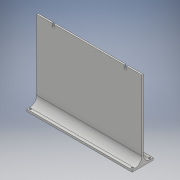
# Autodesk Inventor part: apriltag_body
Saved by Autodesk Inventor 2018 (Build 220112000, 112)
## iProperties
Created: 2020-02-24
Part Number: apriltag_body
Material: Generic
Document SubType Name: Modeling
Designer: bitbots
Density: 1 g/cm^3
Appearance: Default
Author: bitbots
Autodesk Inventor part; units mm, degrees
ref_plane "YZ Plane" through (0, 0, 0) normal (1, 0, 0) x (0, 1, 0)
ref_plane "XZ Plane" through (0, 0, 0) normal (0, 1, 0) x (-1, 0, 0)
ref_plane "XY Plane" through (0, 0, 0) normal (0, 0, 1) x (1, 0, 0)
sketch "Sketch1" plane through (0, 0, 0) normal (0, 1, 0) x (-1, 0, 0)
  line L0 (75, 55) -> (-75, 55)
  line L1 (-75, 55) -> (-75, -55)
  line L2 (-75, -55) -> (75, -55)
  line L3 (75, -55) -> (75, 55)
  line L4 (75, 55) -> (-75, -55) construction
  line L5 (-75, 55) -> (75, -55) construction
  point P0 (0, 0)
  dimension "d0" = 150
  dimension "d1" = 110
  constraints: 12 end point, 2 midpoint, 2 parallel, 1 horizontal, 1 perpendicular
  measures "d0" distance of L2.end L1.end
  measures "d1" distance of L1.end L0.end
extrude "Extrusion1" add sketch "Sketch1" along normal blind 2
sketch "Sketch2" plane through (75, 0, -55) normal (0, 0, -1) x (-1, 0, 0)
  line L0 (0, 0) -> (150, 0) projected
  line L1 (150, 0) -> (150, 2) projected
  line L2 (0, 2) -> (150, 2) projected
  line L3 (0, 0) -> (0, 2) projected
  line L4 (0, 0) -> (0, 2) construction
  line L5 (0, 0) -> (150, 2) construction
  line L6 (150, 0) -> (0, 0) construction
  line L7 (150, 0) -> (0, 2) construction
  line L8 (150, -14) -> (0, -14)
  line L9 (0, -14) -> (0, 16)
  line L10 (0, 16) -> (150, 16)
  line L11 (150, 16) -> (150, -14)
  line L12 (150, -14) -> (0, 16) construction
  line L13 (0, -14) -> (150, 16) construction
  point P0 (75, 0)
  point P1 (75, 1)
  dimension "d4" = 30
  dimension "d5" = 150
  constraints: 16 end point, 3 midpoint, 2 parallel, 1 horizontal, 1 perpendicular
  measures "d4" distance of L8.end L9.end
  measures "d5" distance between parallel lines of L11 L9
extrude "Extrusion2" add sketch "Sketch2" along normal blind 3
fillet "Fillet1" radius 10 2 edges at (0, 0, -55) (0, 2, -55)
sketch "Sketch3" plane through (0, 0, 0) normal (0, -1, 0) x (1, 0, 0)
  line L0 (0, 0) -> (0, 5)
  line L1 (0, 0) -> (5, 0) construction
  line L2 (-50, 55) -> (50, 55)
  line L3 (50, 55) -> (50, -45)
  line L4 (50, -45) -> (-50, -45)
  line L5 (-50, -45) -> (-50, 55)
  line L6 (-50, 55) -> (50, -45) construction
  line L7 (50, 55) -> (-50, -45) construction
  line L8 (-50, 55) -> (-53, 55)
  line L9 (-53, 55) -> (-53, 50)
  line L10 (-53, 50) -> (-50, 50)
  line L11 (-50, 50) -> (-50, 55)
  line L12 (50, 55) -> (53, 55)
  line L13 (53, 55) -> (53, 50)
  line L14 (53, 50) -> (50, 50)
  line L15 (50, 50) -> (50, 55)
  dimension "d9" = 5
  dimension "d10" = 90
  dimension "d11" = 100
  dimension "d12" = 100
  dimension "d13" = 3
  dimension "d14" = 5
  dimension "d15" = 3
  dimension "d16" = 5
  constraints: 32 end point, 6 parallel, 4 horizontal, 4 perpendicular, 2 midpoint, 1 vertical
  measures "d9" distance of L0.start L0.end
  measures "d10" angle of L1 L0
  measures "d11" distance of L3.end L4.end
  measures "d12" distance of L2.end L3.end
  measures "d13" distance of L10.end L9.end
  measures "d14" distance of L9.end L8.end
  measures "d15" distance of L13.end L14.end
  measures "d16" distance of L12.end L13.end
extrude "Extrusion3" cut sketch "Sketch3" against normal up to surface (2 mm away) contours L5 L10 L9 L8 | L12 L13 L14 L3
sketch "Sketch4" plane through (75, 0, -58) normal (0, 0, -1) x (-1, 0, 0)
  line L0 (75, 0) -> (147.5, 0)
  line L1 (0, 0) -> (150, 0) projected
  line L2 (75, 0) -> (147.5, 0) construction
  line L3 (147.5, 0) -> (147.5, -11.5)
  line L4 (150, -10) -> (0, -10) projected
  circle A0 centre (147.5, -11.5) radius 1.35
  line L5 (75, 0) -> (75, -10)
  line L6 (75, 0) -> (85, 0) construction
  circle A1 centre (147.5, 13.5) radius 1.35
  circle A2 centre (2.5, -11.5) radius 1.35
  circle A3 centre (2.5, 13.5) radius 1.35
  line L7 (150, 2) -> (0, 2) projected
  line L8 (75, 0) -> (75, 1)
  line L9 (75, 0) -> (76, 0) construction
  dimension "d19" = 72.5
  dimension "d20" = 0
  dimension "d21" = 11.5
  dimension "d22" = 90
  dimension "d23" = 2.7
  dimension "d24" = 10
  dimension "d25" = 90
  dimension "d28" = 25
  dimension "d31" = 145
  dimension "d34" = 1
  dimension "d35" = 90
  constraints: 14 end point, 4 centre point, 4 horizontal, 3 equal length, 3 perpendicular, 1 coincident, 1 collinear, 1 vertical, 6 other
  measures "d19" distance of L0.start L0.end
  measures "d20" distance between parallel lines of L0 L2
  measures "d21" distance of L0.end L3.end
  measures "d22" angle of L0 L3
  measures "d23" diameter of A0
  measures "d24" distance of L0.start L5.end
  measures "d25" angle of L5 L6
  measures "d28" distance of A0.centre A1.centre
  measures "d31" distance of A0.centre A2.centre
  measures "d34" distance of L0.start L8.end
  measures "d35" angle of L9 L8
extrude "Extrusion4" cut sketch "Sketch4" against normal up to surface (3 mm away) contours A0 | A1 | A2 | A3
body "Solid1"
